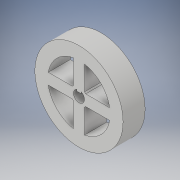
# Autodesk Inventor part: Spokes1
Saved by Autodesk Inventor 2017 (Build 210142000, 142)
## iProperties
Created: 2016-12-01
Part Number: Spokes1
Material: Generic
Document SubType Name: Modeling
Designer: JJ
Density: 1 g/cm^3
Appearance: Default
Author: JJ
Autodesk Inventor part; units mm, degrees
ref_plane "YZ Plane" through (0, 0, 0) normal (1, 0, 0) x (0, 1, 0)
ref_plane "XZ Plane" through (0, 0, 0) normal (0, 1, 0) x (-1, 0, 0)
ref_plane "XY Plane" through (0, 0, 0) normal (0, 0, 1) x (1, 0, 0)
sketch "Sketch1" plane through (0, 0, 0) normal (0, 0, 1) x (1, 0, 0)
  circle A0 centre (0, 0) radius 6.35
  circle A1 centre (0, 0) radius 10
  circle A2 centre (0, 0) radius 50.8
  arc A3 (-35.4016, -6.35) -> (-6.35, -35.4016) centre (0, 0) ccw
  arc A4 (-6.35, 35.4016) -> (-35.4016, 6.35) centre (0, 0) ccw
  arc A5 (35.4016, 6.35) -> (6.35, 35.4016) centre (0, 0) ccw
  arc A6 (6.35, -35.4016) -> (35.4016, -6.35) centre (0, 0) ccw
  line L0 (2.5, 3.9609) -> (-2.5, 3.9609)
  line L1 (-2.5, 3.9609) -> (-2.5, 5.8372)
  line L2 (2.5, 3.9609) -> (2.5, 5.8372)
  arc A7 (-6.35, 35.4016) -> (-35.4016, 6.35) centre (0, 0) ccw
  arc A8 (-6.35, 35.4016) -> (-35.4016, 6.35) centre (0, 0) ccw
  arc A9 (35.4016, 6.35) -> (6.35, 35.4016) centre (0, 0) ccw
  arc A10 (6.35, -35.4016) -> (35.4016, -6.35) centre (0, 0) ccw
  arc A11 (-35.4016, -6.35) -> (-6.35, -35.4016) centre (0, 0) ccw
  arc A12 (6.35, -35.4016) -> (35.4016, -6.35) centre (0, 0) ccw
  line L3 (-35.4016, 6.35) -> (-7.7251, 6.35)
  line L4 (-6.35, 35.4016) -> (-6.35, 7.7251)
  line L5 (6.35, 35.4016) -> (6.35, 7.7251)
  line L6 (35.4016, 6.35) -> (7.7251, 6.35)
  line L7 (35.4016, -6.35) -> (7.7251, -6.35)
  line L8 (6.35, -35.4016) -> (6.35, -7.7251)
  line L9 (-6.35, -35.4016) -> (-6.35, -7.7251)
  line L10 (-35.4016, -6.35) -> (-7.7251, -6.35)
  dimension "d8" = 12.7
  dimension "d22" = 101.6
  constraints: 22 end point, 22 point on circle, 12 centre point, 4 concentric, 3 coincident, 3 parallel, 2 horizontal, 2 perpendicular, 1 point on line, 1 vertical, 10 other
  measures "d8" diameter of A0
  measures "d22" diameter of A2
extrude "Extrusion1" add sketch "Sketch1" along normal blind 25.4 contours L2 L0 L1 A0 | A1 | A2 picked at (0, 4.7573)
body "Solid1"
